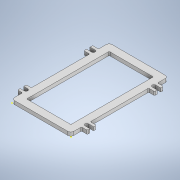
# Autodesk Inventor part: Część5
Saved by Autodesk Inventor 2021 (Build 250183000, 183)
## iProperties
Created: 2023-09-22
Part Number: Część5
Material: Ogólny
Document SubType Name: Modeling
Designer: Jakub
Density: 1 g/cm^3
Appearance: Domyślna
Author: Jakub
Autodesk Inventor part; units mm, degrees
ref_plane "YZ Plane" through (0, 0, 0) normal (1, 0, 0) x (0, 1, 0)
ref_plane "XZ Plane" through (0, 0, 0) normal (0, 1, 0) x (-1, 0, 0)
ref_plane "XY Plane" through (0, 0, 0) normal (0, 0, 1) x (1, 0, 0)
sketch "Szkic1" plane through (0, 0, 0) normal (0, 1, 0) x (-1, 0, 0)
  line L0 (0, 0) -> (-200, 0)
  line L1 (-200, -330) -> (0, -330)
  line L2 (-25, -25) -> (-25, -305)
  line L3 (-25, -305) -> (-175, -305)
  line L4 (-175, -305) -> (-175, -25)
  line L5 (-175, -25) -> (-25, -25)
  line L6 (0, -330) -> (0, -285)
  line L7 (0, -285) -> (-3, -285)
  line L8 (-3, -285) -> (-3, -273)
  line L9 (-3, -273) -> (0, -273)
  line L10 (0, 0) -> (0, -45)
  line L11 (0, -45) -> (-3, -45)
  line L12 (-3, -45) -> (-3, -57)
  line L13 (-3, -57) -> (0, -57)
  line L14 (0, -57) -> (0, -273)
  line L15 (-200, -330) -> (-200, -285)
  line L16 (-200, -285) -> (-197, -285)
  line L17 (-197, -285) -> (-197, -273)
  line L18 (-197, -273) -> (-200, -273)
  line L19 (-200, -273) -> (-200, -264)
  line L20 (-200, -264) -> (-200, -57)
  line L21 (-200, -57) -> (-197, -57)
  line L22 (-197, -57) -> (-197, -45)
  line L23 (-197, -45) -> (-200, -45)
  line L24 (-200, 0) -> (-200, -45)
  line L25 (0, -285) -> (20, -285)
  line L26 (20, -285) -> (20, -294)
  line L27 (20, -294) -> (0, -294)
  line L28 (0, -285) -> (0, -294)
  line L29 (0, -273) -> (20, -273)
  line L30 (20, -273) -> (20, -264)
  line L31 (20, -264) -> (0, -264)
  line L32 (0, -273) -> (0, -264)
  dimension "d0" = 200
  dimension "d1" = 330
  dimension "d2" = 280
  dimension "d3" = 150
  dimension "d40" = 45
  dimension "d41" = 3
  dimension "d42" = 12
  dimension "d43" = 45
  dimension "d44" = 3
  dimension "d45" = 12
  dimension "d46" = 3
  dimension "d47" = 12
  dimension "d48" = 9
  dimension "d49" = 3
  dimension "d50" = 12
  dimension "d55" = 20
  dimension "d56" = 9
  dimension "d57" = 9
  constraints: 66 end point, 18 perpendicular, 12 point on line, 3 horizontal, 3 vertical, 2 collinear
  measures "d0" distance of L0.start L0.end
  measures "d1" distance of L0.end L1.start
  measures "d2" distance of L2.start L2.end
  measures "d3" distance of L2.end L3.end
  measures "d40" distance of L1.end L6.end
  measures "d41" distance of L6.end L7.end
  measures "d42" distance of L7.end L8.end
  measures "d43" distance of L0.start L10.end
  measures "d44" distance of L10.end L11.end
  measures "d45" distance of L11.end L12.end
  measures "d46" distance of L15.end L16.end
  measures "d47" distance of L16.end L17.end
  measures "d48" distance of L18.end L19.end
  measures "d49" distance of L20.end L21.end
  measures "d50" distance of L21.end L22.end
  measures "d55" distance of L6.end L25.end
  measures "d56" distance of L25.end L26.end
  measures "d57" distance of L29.end L30.end
extrude "Wyciągnięcie proste1" add sketch "Szkic1" along normal blind 12 contours L10 L11 L12 L13 L14 L9 L8 L7 L6 L1 L15 L16 L17 L18 L19 L20 L21 L22 L23 L24 L0
fillet "Zaokrąglenie1" radius 3 1 edges at (25, 6, -305)
fillet "Zaokrąglenie2" radius 3 1 edges at (175, 6, -305)
fillet "Zaokrąglenie3" radius 3 1 edges at (175, 6, -25)
fillet "Zaokrąglenie4" radius 3 1 edges at (25, 6, -25)
fillet "Zaokrąglenie5" radius 10 1 edges at (0, 6, 0)
fillet "Zaokrąglenie6" radius 10 1 edges at (200, 6, 0)
fillet "Zaokrąglenie7" radius 10 1 edges at (200, 6, -330)
fillet "Zaokrąglenie8" radius 10 1 edges at (0, 6, -330)
sketch "Szkic8" plane through (0, 0, 0) normal (0, 1, 0) x (-1, 0, 0)
  line L0 (-3, -54) -> (-3, -74)
  line L1 (-3, -74) -> (-3, -34)
  line L2 (-3, -34) -> (-9, -34)
  line L3 (-9, -34) -> (-9, -74)
  line L4 (-9, -74) -> (-3, -74)
  line L5 (-3, -66) -> (17, -66)
  line L6 (17, -66) -> (17, -57)
  line L7 (17, -57) -> (-3, -57)
  line L8 (-3, -57) -> (-3, -45)
  line L9 (-3, -45) -> (17, -45)
  line L10 (17, -45) -> (17, -36)
  line L11 (17, -36) -> (-3, -36)
  line L12 (-3, -34) -> (-3, -29)
  line L13 (-3, -29) -> (-9, -29)
  line L14 (-9, -29) -> (-9, -34)
  point P0 (0, 0)
  dimension "d23" = 20
  dimension "d24" = 40
  dimension "d25" = 6
  dimension "d26" = 20
  dimension "d27" = 9
  dimension "d28" = 12
  dimension "d29" = 20
  dimension "d30" = 9
  dimension "d31" = 5
  constraints: 30 end point, 8 point on line, 6 perpendicular, 2 vertical, 1 collinear, 1 parallel
  measures "d23" distance of L0.start L0.end
  measures "d24" distance of L0.end L1.end
  measures "d25" distance of L1.end L2.end
  measures "d26" distance of L5.start L5.end
  measures "d27" distance of L5.end L6.end
  measures "d28" distance of L7.end L8.end
  measures "d29" distance of L8.end L9.end
  measures "d30" distance of L9.end L10.end
  measures "d31" distance of L1.end L12.end
extrude "Wyciągnięcie proste2" add sketch "Szkic8" along normal blind 12
fillet "Zaokrąglenie12" radius 3 1 edges at (-17, 6, -66)
fillet "Zaokrąglenie13" radius 3 1 edges at (-17, 6, -36)
fillet "Zaokrąglenie15" radius 6 1 edges at (3, 6, -45)
fillet "Zaokrąglenie16" radius 6 1 edges at (3, 6, -57)
fillet "Zaokrąglenie17" radius 3 1 edges at (0, 6, -66)
fillet "Zaokrąglenie18" radius 3 1 edges at (0, 6, -36)
sketch "Szkic10" plane through (0, 0, -273) normal (-1, 0, 0) x (0, 0, 1)
  point P0 (273, 0)
sketch "Szkic11" plane through (0, 12, 0) normal (0, 1, 0) x (1, 0, 0)
  line L0 (0, 273) -> (0, 69) projected
  line L1 (0, 273) -> (-20, 273)
  line L2 (-20, 273) -> (-20, 264)
  line L3 (-20, 264) -> (0, 264)
  point P0 (0, 0)
  dimension "d58" = 20
  dimension "d59" = 9
  constraints: 6 end point, 2 perpendicular, 1 horizontal, 1 point on line
  measures "d58" distance of L0.start L1.end
  measures "d59" distance of L1.end L2.end
sketch "Szkic12" plane through (0, 12, 0) normal (0, 1, 0) x (1, 0, 0)
  line L0 (0, 285) -> (-20, 285)
  line L1 (-20, 285) -> (-20, 294)
  line L2 (-20, 294) -> (0, 294)
  line L3 (0, 320) -> (0, 285) projected
  point P0 (0, 0)
  dimension "d60" = 20
  dimension "d61" = 9
  constraints: 6 end point, 2 perpendicular, 1 horizontal, 1 point on line
  measures "d60" distance of L0.start L0.end
  measures "d61" distance of L0.end L1.end
extrude "Wyciągnięcie proste3" add sketch "Szkic11" against normal blind 12
extrude "Wyciągnięcie proste4" add sketch "Szkic12" against normal blind 12
sketch "Szkic13" plane through (0, 12, 0) normal (0, 1, 0) x (1, 0, 0)
  line L0 (200, 10) -> (200, 45) projected
  line L1 (200, 45) -> (200, 36)
  line L2 (200, 36) -> (220, 36)
  line L3 (220, 36) -> (220, 45)
  line L4 (220, 45) -> (200, 45)
  line L5 (197, 57) -> (200, 57) projected
  line L6 (200, 57) -> (200, 66)
  line L7 (200, 57) -> (200, 273) projected
  line L8 (200, 66) -> (220, 66)
  line L9 (220, 66) -> (220, 57)
  line L10 (200, 57) -> (220, 57)
  point P0 (0, 0)
  dimension "d66" = 9
  dimension "d67" = 20
  dimension "d68" = 9
  dimension "d69" = 9
  constraints: 16 end point, 4 point on line, 3 perpendicular, 1 horizontal
  measures "d66" distance of L0.end L1.end
  measures "d67" distance of L1.end L2.end
  measures "d68" distance of L2.end L3.end
  measures "d69" distance of L5.end L6.end
extrude "Wyciągnięcie proste5" add sketch "Szkic13" against normal blind 12
sketch "Szkic14" plane through (200, 0, -273) normal (1, 0, 0) x (0, 0, -1)
  point P0 (-273, 0)
sketch "Szkic15" plane through (0, 12, 0) normal (0, 1, 0) x (1, 0, 0)
  line L0 (200, 66) -> (200, 273) projected
  line L1 (200, 273) -> (220, 273)
  line L2 (220, 273) -> (220, 264)
  line L3 (220, 264) -> (200, 264)
  point P0 (0, 0)
  dimension "d72" = 20
  dimension "d73" = 9
  constraints: 6 end point, 2 perpendicular, 1 horizontal, 1 point on line
  measures "d72" distance of L0.end L1.end
  measures "d73" distance of L1.end L2.end
sketch "Szkic16" plane through (200, 0, -285) normal (1, 0, 0) x (0, 0, -1)
  point P0 (-285, 0)
sketch "Szkic17" plane through (0, 12, 0) normal (0, 1, 0) x (1, 0, 0)
  line L0 (197, 285) -> (200, 285) projected
  line L1 (200, 285) -> (200, 265)
  line L2 (200, 285) -> (200, 320) projected
  line L3 (200, 285) -> (220, 285)
  line L4 (220, 285) -> (220, 294)
  line L5 (220, 294) -> (200, 294)
  line L6 (200, 294) -> (200, 285)
  point P0 (0, 0)
  dimension "d74" = 20
  dimension "d75" = 20
  dimension "d76" = 9
  dimension "d77" = 20
  constraints: 10 end point, 2 collinear, 2 perpendicular, 1 point on line
  measures "d74" distance of L0.end L1.end
  measures "d75" distance of L0.end L3.end
  measures "d76" distance of L3.end L4.end
  measures "d77" distance of L4.end L5.end
extrude "Wyciągnięcie proste6" add sketch "Szkic15" against normal blind 12
extrude "Wyciągnięcie proste7" add sketch "Szkic17" against normal blind 12
fillet "Zaokrąglenie19" radius 6 1 edges at (197, 6, -273)
fillet "Zaokrąglenie20" radius 6 1 edges at (197, 6, -285)
fillet "Zaokrąglenie21" radius 6 1 edges at (197, 6, -45)
fillet "Zaokrąglenie22" radius 6 1 edges at (197, 6, -57)
fillet "Zaokrąglenie23" radius 6 1 edges at (3, 6, -273)
fillet "Zaokrąglenie24" radius 6 1 edges at (3, 6, -285)
fillet "Zaokrąglenie25" radius 3 1 edges at (0, 6, -294)
fillet "Zaokrąglenie26" radius 3 1 edges at (-20, 6, -294)
fillet "Zaokrąglenie27" radius 3 1 edges at (-20, 6, -264)
fillet "Zaokrąglenie28" radius 3 1 edges at (0, 6, -264)
fillet "Zaokrąglenie29" radius 3 1 edges at (200, 6, -66)
fillet "Zaokrąglenie30" radius 3 1 edges at (220, 6, -66)
fillet "Zaokrąglenie31" radius 3 1 edges at (220, 6, -36)
fillet "Zaokrąglenie32" radius 3 1 edges at (200, 6, -36)
fillet "Zaokrąglenie33" radius 3 1 edges at (200, 6, -264)
fillet "Zaokrąglenie34" radius 3 1 edges at (220, 6, -264)
fillet "Zaokrąglenie35" radius 3 1 edges at (220, 6, -294)
fillet "Zaokrąglenie36" radius 3 1 edges at (200, 6, -294)
